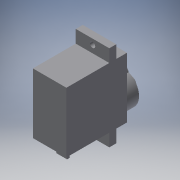
# Autodesk Inventor part: Servo
Saved by Autodesk Inventor 2017 (Build 210142000, 142)
## iProperties
Created: 2020-08-23
Part Number: Servo
Material: Generic
Document SubType Name: Modeling
Designer: agustin
Density: 1 g/cm^3
Appearance: Default
Author: agustin
Autodesk Inventor part; units mm, degrees
ref_plane "YZ Plane" through (0, 0, 0) normal (1, 0, 0) x (0, 1, 0)
ref_plane "XZ Plane" through (0, 0, 0) normal (0, 1, 0) x (-1, 0, 0)
ref_plane "XY Plane" through (0, 0, 0) normal (0, 0, 1) x (1, 0, 0)
sketch "Sketch1" plane through (0, 0, 0) normal (0, 1, 0) x (-1, 0, 0)
  line L0 (12.5, 22.5) -> (-12.5, 22.5)
  line L1 (-12.5, 22.5) -> (-12.5, -22.5)
  line L2 (-12.5, -22.5) -> (12.5, -22.5)
  line L3 (12.5, -22.5) -> (12.5, 22.5)
  line L4 (12.5, 22.5) -> (-12.5, -22.5) construction
  line L5 (-12.5, 22.5) -> (12.5, -22.5) construction
  point P0 (0, 0)
  dimension "d0" = 25
  dimension "d1" = 45
  constraints: 12 end point, 2 midpoint, 2 parallel, 1 horizontal, 1 perpendicular
  measures "d0" distance of L2.end L1.end
  measures "d1" distance of L1.end L0.end
extrude "Extrusion1" add sketch "Sketch1" along normal blind 32
sketch "Sketch2" plane through (0, 32, 0) normal (0, 1, 0) x (1, 0, 0)
  line L0 (12.5, -32) -> (-12.5, -32)
  line L1 (-12.5, -32) -> (-12.5, 32)
  line L2 (-12.5, 32) -> (12.5, 32)
  line L3 (12.5, 32) -> (12.5, -32)
  line L4 (12.5, -32) -> (-12.5, 32) construction
  line L5 (-12.5, -32) -> (12.5, 32) construction
  line L6 (0, -32) -> (0, -28)
  line L7 (0, 32) -> (0, 28)
  circle A0 centre (0, -28) radius 2
  circle A1 centre (0, 28) radius 2
  point P0 (0, 0)
  dimension "d4" = 64
  dimension "d5" = 4
  dimension "d6" = 4
  dimension "d7" = 4
  dimension "d8" = 4
  constraints: 16 end point, 4 midpoint, 2 centre point, 2 coincident, 2 parallel, 2 vertical, 1 horizontal, 1 perpendicular
  measures "d4" distance of L0.end L1.end
  measures "d5" distance of L6.start L6.end
  measures "d6" distance of L7.start L7.end
  measures "d7" diameter of A0
  measures "d8" diameter of A1
extrude "Extrusion2" add sketch "Sketch2" along normal blind 5.2
sketch "Sketch3" plane through (0, 37.2, 0) normal (0, 1, 0) x (1, 0, 0)
  line L0 (12.5, 22.5) -> (-12.5, 22.5) projected
  line L1 (-12.5, -22.5) -> (12.5, -22.5)
  line L2 (12.5, -22.5) -> (12.5, 22.5)
  line L3 (12.5, 22.5) -> (-12.5, 22.5)
  line L4 (-12.5, 22.5) -> (-12.5, -22.5)
  line L5 (-12.5, -22.5) -> (12.5, 22.5) construction
  line L6 (12.5, -22.5) -> (-12.5, 22.5) construction
  point P0 (0, 0)
  constraints: 12 end point, 2 midpoint, 2 parallel, 1 horizontal, 1 perpendicular
extrude "Extrusion3" add sketch "Sketch3" along normal blind 8
sketch "Sketch4" plane through (0, 45.2, 0) normal (0, 1, 0) x (1, 0, 0)
  line L0 (-12.5, 22.5) -> (-12.5, -22.5) projected
  line L1 (12.5, 22.5) -> (-12.5, 22.5) projected
  line L2 (12.5, -22.5) -> (12.5, 22.5) projected
  arc A0 (4.7196, -1.5748) -> (-4.7196, -1.5748) centre (0, 10) ccw
  line L3 (-12.5, 22.5) -> (12.5, 22.5) projected
  arc A1 (-4.7196, -1.5748) -> (4.7196, -1.5748) centre (0, -0.7) ccw
  point P0 (0, 0)
  constraints: 4 point on circle, 3 tangent, 2 centre point
extrude "Extrusion4" add sketch "Sketch4" along normal blind 9 contours A0 A1
sketch "Sketch5" plane through (0, 54.2, 0) normal (0, 1, 0) x (1, 0, 0)
  arc A0 (4.7196, -1.5748) -> (-4.7196, -1.5748) centre (0, 10) ccw projected
  circle A1 centre (0, 10) radius 4.5
  point P0 (0, 0)
  dimension "d18" = 9
  constraints: 1 centre point, 1 coincident
  measures "d18" diameter of A1
extrude "Extrusion5" add sketch "Sketch5" along normal blind 6
sketch "Sketch6" plane through (12.5, 0, -22.5) normal (0, 0, -1) x (-1, 0, 0)
  line L0 (8.5, 11) -> (16.5, 11)
  line L1 (16.5, 11) -> (16.5, 9)
  line L2 (16.5, 9) -> (8.5, 9)
  line L3 (8.5, 9) -> (8.5, 11)
  line L4 (8.5, 11) -> (16.5, 9) construction
  line L5 (16.5, 11) -> (8.5, 9) construction
  point P0 (12.5, 0)
  dimension "d22" = 8
  dimension "d23" = 2
  constraints: 12 end point, 2 parallel, 1 horizontal, 1 perpendicular
  measures "d22" distance of L1.end L2.end
  measures "d23" distance of L0.end L1.end
extrude "Extrusion6" add sketch "Sketch6" along normal blind 10
scale "Scale1" factors (0.5, 0.5, 0.5) then translate (6.25, 8, -11.25) bodies 1
body "Solid1"
